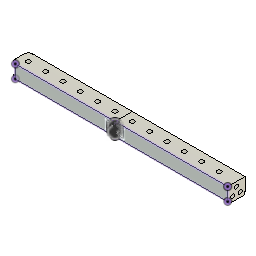
entire pole assembly (Autodesk Fusion 360 design; units mm, degrees)
Autodesk Fusion 360 part; units mm, degrees
sketch "Sketch1" plane through (0, 0, 0) normal (0, 0, 1) x (1, 0, 0)
  line L0 (0, 10) -> (0, -10)
  line L1 (0, -10) -> (-250, -10)
  line L2 (-250, -10) -> (-250, 10)
  line L3 (-250, 10) -> (0, 10)
  line L4 (0, -10) -> (-250, 10) construction
  line L5 (-250, -10) -> (0, 10) construction
  point P0 (-125, 0)
  point P1 (-250, 0)
  dimension "d1" = 20
  dimension "d36" = 250
  constraint perpendicular L0 L1
  constraint parallel L0 L2
  constraint parallel L1 L3
  constraint vertical L0
  constraint midpoint L4 P0
  constraint horizontal origin P0
  constraint coincident origin L0
  constraint midpoint L2 P1
  measures "d1" distance of L0.start L0.end
  measures "d36" distance of origin P1
extrude "Extrude1" add sketch "Sketch1" along normal blind 18 makes body 1
sketch "Sketch2" plane through (0, 0, 18) normal (0, 0, 1) x (-1, 0, 0)
  line L0 (250, -10) -> (250, 10)
  line L1 (250, 10) -> (0, 10)
  line L2 (0, 10) -> (0, -10)
  line L3 (0, -10) -> (250, -10)
  circle A0 centre (280, 0) radius 2
  circle A1 centre (260, 0) radius 2
  circle A2 centre (240, 0) radius 2
  circle A3 centre (220, 0) radius 2
  circle A4 centre (200, 0) radius 2
  circle A5 centre (180, 0) radius 2
  circle A6 centre (160, 0) radius 2
  circle A7 centre (140, 0) radius 2
  circle A8 centre (120, 0) radius 2
  circle A9 centre (100, 0) radius 2
  circle A10 centre (80, 0) radius 2
  circle A11 centre (60, 0) radius 2
  circle A12 centre (40, 0) radius 2
  circle A13 centre (20, 0) radius 2
  point P0 (20, 0)
  point P1 (40, 0)
  point P2 (60, 0)
  point P3 (80, 0)
  point P4 (100, 0)
  point P5 (120, 0)
  point P6 (140, 0)
  point P7 (160, 0)
  point P8 (180, 0)
  point P9 (200, 0)
  point P10 (220, 0)
  point P11 (240, 0)
  point P12 (260, 0)
  point P13 (280, 0)
  dimension "d9" = 20
  dimension "d10" = 0
  dimension "d11" = 4
  dimension "d12" = 4
  dimension "d13" = 4
  dimension "d14" = 4
  dimension "d15" = 4
  dimension "d16" = 4
  dimension "d17" = 4
  dimension "d18" = 4
  dimension "d19" = 4
  dimension "d20" = 4
  dimension "d21" = 4
  dimension "d22" = 4
  dimension "d23" = 4
  dimension "d24" = 4
  constraint coincident P13 A0.centre
  constraint coincident P12 A1.centre
  constraint coincident P11 A2.centre
  constraint coincident P10 A3.centre
  constraint coincident P9 A4.centre
  constraint coincident P8 A5.centre
  constraint coincident P7 A6.centre
  constraint coincident P6 A7.centre
  constraint coincident P5 A8.centre
  constraint coincident P4 A9.centre
  constraint coincident P3 A10.centre
  constraint coincident P2 A11.centre
  constraint coincident P1 A12.centre
  measures "d11" diameter of A0
  measures "d12" diameter of A1
  measures "d13" diameter of A2
  measures "d14" diameter of A3
  measures "d15" diameter of A4
  measures "d16" diameter of A5
  measures "d17" diameter of A6
  measures "d18" diameter of A7
  measures "d19" diameter of A8
  measures "d20" diameter of A9
  measures "d21" diameter of A10
  measures "d22" diameter of A11
  measures "d23" diameter of A12
  measures "d24" diameter of A13
extrude "Extrude2" cut sketch "Sketch2" against normal blind 90 contours A0 | A1 | A2 | A3 | A4 | A5 | A6 | A7 | A8 | A9 | A10 | A11 | A12 | A13 bodies 1
fillet "Fillet1" radius 3 2 edges at (-125, -10, 0) (-125, 10, 0) on bodies 1
sketch "Sketch3" plane through (0, 0, 0) normal (1, 0, 0) x (0, 1, 0)
  arc A0 (7, 0) -> (10, 3) centre (7, 3) ccw
  line L0 (10, 3) -> (10, 18)
  line L1 (10, 18) -> (-10, 18)
  line L2 (-10, 18) -> (-10, 3)
  arc A1 (-10, 3) -> (-7, 0) centre (-7, 3) ccw
  line L3 (-7, 0) -> (7, 0)
  line L4 (0, 36) -> (0, 0) construction
  line L5 (0, 13.008) -> (-4.337, 5.496) construction
  line L6 (-4.337, 5.496) -> (4.337, 5.496) construction
  line L7 (4.337, 5.496) -> (0, 13.008) construction
  circle A2 centre (0, 13.008) radius 2.25
  circle A3 centre (4.337, 5.496) radius 2.25
  circle A4 centre (-4.337, 5.496) radius 2.25
  point P0 (0, 18)
  point P1 (0, 8)
  dimension "d29" = 8.6741
  dimension "d30" = 8
  dimension "d31" = 4.5
  dimension "d32" = 4.5
  dimension "d33" = 4.5
  constraint midpoint L4 P0
  constraint coincident L1 P0
  constraint coincident L4.end origin
  constraint perpendicular L3 L4
  constraint coincident L4 P1
  constraint coincident L4 L5.start
  constraint coincident L5.start L7.end
  constraint coincident L6.end L7.start
  constraint coincident L5.end L6.start
  measures "d29" distance of L5.end L6.end
  measures "d30" distance of L4.end P1
  measures "d31" diameter of A2
  measures "d32" diameter of A3
  measures "d33" diameter of A4
extrude "Extrude3" cut sketch "Sketch3" against normal blind 5.5 contours A2 | A3 | A4 bodies 1
sketch "Sketch4" plane through (0, -10, 0) normal (0, -1, 0) x (1, 0, 0)
  line L0 (-250, 3) -> (0, 3)
  line L1 (0, 3) -> (0, 18)
  line L2 (0, 18) -> (-250, 18)
  line L3 (-250, 18) -> (-250, 3)
fillet "Fillet2" radius 5 5 edges at (-250, 10, 10.5) (-250, 9.1213, 0.8787) (-250, 0, 0) (-250, -9.1213, 0.8787) (-250, -10, 10.5) on bodies 1
ref_plane "WorkPlane1" through (-130, 0, 9) normal (1, 0, 0) x (0, 1, 0)
split "Split1" by plane through (-130, 0, 9) normal (1, 0, 0) bodies 1 makes body 2 at (-6, 0, 18)
sketch "Sketch5" plane through (0, -10, 0) normal (0, -1, 0) x (1, 0, 0)
  line L0 (-130, 3) -> (-130, 18)
  line L1 (-130, 18) -> (-245, 18)
  line L2 (-245, 18) -> (-245, 3)
  line L3 (-245, 3) -> (-130, 3)
  line L4 (-130, 18) -> (-130, 3)
  line L5 (-130, 3) -> (0, 3)
  line L6 (0, 3) -> (0, 18)
  line L7 (0, 18) -> (-130, 18)
  line L8 (-120, 15.5) -> (-140, 15.5) construction
  line L9 (-140, 15.5) -> (-140, 5.5) construction
  line L10 (-140, 5.5) -> (-120, 5.5) construction
  line L11 (-120, 5.5) -> (-120, 15.5) construction
  line L12 (-120, 15.5) -> (-140, 5.5) construction
  line L13 (-140, 15.5) -> (-120, 5.5) construction
  line L14 (-120, 5.5) -> (-120, 15.5)
  line L15 (-130, 13.5) -> (-140, 15.5)
  line L16 (-140, 5.5) -> (-140, 15.5)
  line L17 (-140, 5.5) -> (-130, 7.5)
  line L18 (-130, 7.5) -> (-120, 5.5)
  line L19 (-130, 13.5) -> (-120, 15.5)
  point P0 (-130, 10.5)
  point P1 (-130, 10.5)
  dimension "d41" = 20
  dimension "d42" = 10
  dimension "d43" = 3
  dimension "d44" = 3
  constraint midpoint L4 P1
  constraint horizontal L8
  constraint perpendicular L8 L9
  constraint parallel L8 L10
  constraint parallel L9 L11
  constraint coincident L12 P1
  constraint coincident L13 P1
  constraint coincident P1 P0
  constraint coincident L4 L15.start
  constraint coincident L4 L17.end
  measures "d41" distance of L9.end L10.end
  measures "d42" distance of L8.end L9.end
  measures "d43" distance of P1 L15.start
  measures "d44" distance of P1 L17.end
move_face "OffsetFaces1" offset -0.5 12 faces at (-21.9901, 0.1991, 12) (-41.9901, 0.1991, 12) (-61.9901, 0.1991, 12) (-78.4679, -1.2856, 6) (-98.6766, -1.4996, 12) (-118.6766, -1.4996, 12) (-141.1675, -1.6239, 6) (-161.1675, -1.6239, 6) (-181.1675, -1.6239, 6) (-199.0876, 1.7797, 12) (-221.1675, -1.6239, 6) (-239.0876, 1.7797, 12) on bodies 1 2
extrude "Extrude4" cut sketch "Sketch5" against normal blind 4 contours L0 L4 L15 L16 L17 | L0 L4 L14 L18 L19 bodies 1 2
extrude "Extrude5" cut sketch "Sketch5" along normal blind 4 from surface at -20 contours L0 L4 L15 L16 L17 | L0 L4 L14 L18 L19 bodies 1 2
extrude "Extrude6" add sketch "Sketch5" against normal blind 4 separate body contours L0 L4 L15 L16 L17 | L0 L4 L14 L18 L19 makes body 3
chamfer "Chamfer1" distance 0.3 angle 45 1 faces at (-136.6667, -6, 11.5) tangent chain off on bodies 3
move_face "OffsetFaces2" offset -0.1 6 faces at (-123.3333, -7.5333, 14.8333) (-136.6667, -7.5333, 14.8333) (-140, -7.5333, 12.1667) (-136.6667, -8.7667, 6.1667) (-126.6667, -8.7667, 6.8333) (-120, -7.5333, 12.1667) on bodies 3
equation "supportheight = 300"
named bodies: "pole section 1", "pole section 2", "bowtie connector"
